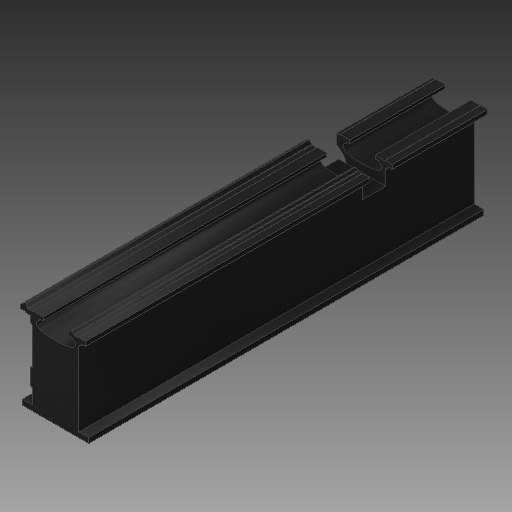
# Autodesk Inventor part: BED
Saved by Autodesk Inventor 2018 (Build 220112000, 112)
## iProperties
Created: 2017-02-14
Part Number: BED
Material: Iron, Cast
Document SubType Name: Modeling
Designer: M228540
Density: 7.15 g/cm^3
Appearance: Black Cast
Author: M228540
Autodesk Inventor part; units mm, degrees
ref_plane "YZ Plane" through (0, 0, 0) normal (1, 0, 0) x (0, 1, 0)
ref_plane "XZ Plane" through (0, 0, 0) normal (0, 1, 0) x (-1, 0, 0)
ref_plane "XY Plane" through (0, 0, 0) normal (0, 0, 1) x (1, 0, 0)
sketch "Sketch1" plane through (0, 0, 0) normal (0, 0, 1) x (1, 0, 0)
  line L0 (11.5989, 4.8072) -> (2.0726, 10.3072)
  line L1 (11.5989, 4.8072) -> (22.5989, 4.8072) construction
  line L2 (2.0726, 10.3072) -> (-7.9274, 10.3072)
  line L3 (-7.9274, 10.3072) -> (-7.9274, 22.0072)
  line L4 (-7.9274, 22.0072) -> (0.1717, 31.6594)
  line L5 (0.1717, 31.6594) -> (3.9717, 31.6594)
  line L6 (3.9717, 31.6594) -> (11.7854, 25.103)
  line L7 (11.7854, 25.103) -> (11.7854, 21.903)
  line L8 (11.7854, 21.903) -> (27.8854, 21.903)
  line L9 (27.8854, 21.903) -> (27.8854, 23.903)
  line L10 (27.8854, 23.903) -> (53.0854, 23.903)
  line L11 (53.0854, 23.903) -> (53.0854, 8.203)
  line L12 (53.0854, 8.203) -> (38.3854, 8.203)
  line L13 (38.3854, 8.203) -> (38.3854, 0.203) construction
  line L14 (38.3854, 0.203) -> (33.7666, 0.203) construction
  line L15 (38.3854, 8.203) -> (33.7666, 0.203)
  line L16 (38.3854, 8.203) -> (62.019, 8.203) construction
  line L17 (33.7666, 0.203) -> (33.7666, -3.797) construction
  arc A0 (33.7666, 0.203) -> (29.7666, -3.797) centre (33.7666, -3.797) ccw
  line L18 (29.7666, -3.797) -> (29.7666, -65.797)
  line L19 (29.7666, -65.797) -> (29.7666, -269.797)
  line L20 (-7.9274, 10.3072) -> (84.2692, 10.3072) construction
  line L21 (-100.122, 11.3032) -> (-98.5294, 23.903)
  line L22 (-98.5294, 23.903) -> (-134.7294, 23.903)
  line L23 (-98.5294, 23.903) -> (-62.3294, 23.903) construction
  line L24 (-134.7294, 23.903) -> (-134.7294, 21.903)
  line L25 (-134.7294, 21.903) -> (-153.7294, 21.903)
  line L26 (-153.7294, 21.903) -> (-153.7294, 23.903)
  line L27 (-153.7294, 23.903) -> (-162.2142, 34.0148)
  line L28 (-162.2142, 34.0148) -> (-166.8142, 34.0148)
  line L29 (-166.8142, 34.0148) -> (-179.0709, 23.7302)
  line L30 (-179.0709, 23.7302) -> (-179.0709, 9.7302)
  line L31 (-179.0709, 9.7302) -> (-165.0709, 9.7302)
  line L32 (-165.0709, 9.7302) -> (-165.0709, 6.7302) construction
  line L33 (-165.0709, 6.7302) -> (-163.3389, 6.7302) construction
  line L34 (-165.0709, 9.7302) -> (-163.3389, 6.7302)
  line L35 (-165.0709, 9.7302) -> (-161.6857, 9.7302) construction
  line L36 (-163.3389, 6.7302) -> (-145.9389, 6.7302)
  line L37 (-145.9389, 6.7302) -> (-145.9389, -15.7698)
  line L38 (-145.9389, -15.7698) -> (-145.9389, -22.7698) construction
  arc A1 (-138.9389, -22.7698) -> (-145.9389, -15.7698) centre (-145.9389, -22.7698) ccw
  line L39 (-138.9389, -22.7698) -> (-138.9389, -157.2698)
  line L40 (-138.9389, -22.7698) -> (-4.4389, -22.7698) construction
  line L41 (-138.9389, -157.2698) -> (-145.9389, -157.2698)
  line L42 (-145.9389, -157.2698) -> (-145.9389, -212.7698)
  line L43 (-145.9389, -212.7698) -> (-138.9389, -212.7698)
  line L44 (-138.9389, -212.7698) -> (-138.9389, -269.797)
  line L45 (-138.9389, -22.7698) -> (-145.9389, -22.7698) construction
  line L46 (29.7666, -3.797) -> (33.7666, -3.797) construction
  line L47 (-138.9389, -269.797) -> (-173.9389, -269.797)
  line L48 (-138.9389, -269.797) -> (-103.9389, -269.797) construction
  line L49 (-173.9389, -269.797) -> (-173.9389, -287.797)
  line L50 (29.7666, -269.797) -> (64.7666, -269.797)
  line L51 (29.7666, -269.797) -> (64.7666, -269.797) construction
  line L52 (64.7666, -269.797) -> (64.7666, -287.797)
  line L53 (64.7666, -287.797) -> (-173.9389, -287.797)
  line L54 (-100.122, 11.3032) -> (-110.722, 11.3032)
  line L55 (-100.122, 11.3032) -> (-89.522, 11.3032) construction
  line L56 (-110.722, 11.3032) -> (-114.722, 4.375)
  line L57 (-114.722, 4.375) -> (-119.5625, 1.8016) construction
  line L58 (-119.5625, 1.8016) -> (-124.3659, -3.6968) construction
  line L59 (-124.3659, -3.6968) -> (-125.2502, -13.8603) construction
  line L60 (-125.2502, -13.8603) -> (-112.722, -24.0101) construction
  line L61 (-112.722, -24.0101) -> (-52.4666, -30.3406) construction
  line L62 (-52.4666, -30.3406) -> (0.1681, -22.7698) construction
  line L63 (0.1681, -22.7698) -> (13.3927, -16.0523) construction
  line L64 (13.3927, -16.0523) -> (19.8318, -4.9385) construction
  line L65 (19.8318, -4.9385) -> (14.7145, 3.0084) construction
  line L66 (14.7145, 3.0084) -> (11.5989, 4.8072) construction
  spline S0 degree 4 poles (-114.722, 4.375) (-119.5625, 1.8016) (-124.3659, -3.6968) (-125.2502, -13.8603) (-112.722, -24.0101) (-52.4666, -30.3406) (0.1681, -22.7698) (13.3927, -16.0523) (19.8318, -4.9385) (14.7145, 3.0084) (11.5989, 4.8072) knots 0 0 0 0 0 1 2 3 4 5 6 7 7 7 7 7
  point P0 (0, 0)
  dimension "d0" = 11
  dimension "d1" = 150
  dimension "d2" = 10
  dimension "d3" = 11.7
  dimension "d4" = 12.6
  dimension "d5" = 140
  dimension "d6" = 3.8
  dimension "d7" = 10.2
  dimension "d8" = 140
  dimension "d9" = 3.2
  dimension "d10" = 16.1
  dimension "d11" = 2
  dimension "d12" = 25.2
  dimension "d13" = 15.7
  dimension "d14" = 14.7
  dimension "d15" = 8
  dimension "d16" = 120
  dimension "d17" = 4
  dimension "d18" = 62
  dimension "d19" = 204
  dimension "d22" = 92.2
  dimension "d24" = 12.7
  dimension "d25" = 36.2
  dimension "d26" = 180
  dimension "d27" = 2
  dimension "d28" = 19
  dimension "d29" = 2
  dimension "d30" = 13.2
  dimension "d31" = 140
  dimension "d32" = 4.6
  dimension "d33" = 16
  dimension "d34" = 140
  dimension "d35" = 14
  dimension "d36" = 14
  dimension "d37" = 90
  dimension "d38" = 3
  dimension "d39" = 60
  dimension "d40" = 17.4
  dimension "d41" = 22.5
  dimension "d43" = 134.5
  dimension "d44" = 90
  dimension "d46" = 55.5
  dimension "d47" = 90
  dimension "d50" = 90
  dimension "d51" = 35
  dimension "d52" = 180
  dimension "d53" = 18
  dimension "d54" = 90
  dimension "d55" = 35
  dimension "d57" = 18
  dimension "d59" = 180
  dimension "d60" = 8
  dimension "d61" = 120
  dimension "d62" = 62
  dimension "d98" = 7
  dimension "d103" = 7
  constraints: 114 end point, 22 perpendicular, 19 horizontal, 6 equal length, 5 vertical, 4 point on circle, 4 point on line, 2 centre point, 2 coincident, 2 parallel, 1 collinear, 3 other
  measures "d0" distance of L0.start L0.end
  measures "d1" angle of L1 L0
  measures "d2" distance of L0.end L2.end
  measures "d3" distance of L2.end L3.end
  measures "d4" distance of L3.end L4.end
  measures "d5" angle of L3 L4
  measures "d6" distance of L4.end L5.end
  measures "d7" distance of L5.end L6.end
  measures "d8" angle of L5 L6
  measures "d9" distance of L6.end L7.end
  measures "d10" distance of L7.end L8.end
  measures "d11" distance of L8.end L9.end
  measures "d12" distance of L9.end L10.end
  measures "d13" distance of L10.end L11.end
  measures "d14" distance of L11.end L12.end
  measures "d15" distance of L12.end L13.end
  measures "d16" angle of L15 L16
  measures "d17" distance of L14.end L17.end
  measures "d18" distance of L18.start L18.end
  measures "d19" distance of L18.end L19.end
  measures "d22" distance of L2.end L21.start
  measures "d24" distance of L21.start L21.end
  measures "d25" distance of L21.end L22.end
  measures "d26" angle of L22 L23
  measures "d27" distance of L22.end L24.end
  measures "d28" distance of L24.end L25.end
  measures "d29" distance of L25.end L26.end
  measures "d30" distance of L26.end L27.end
  measures "d31" angle of L27 L26
  measures "d32" distance of L27.end L28.end
  measures "d33" distance of L28.end L29.end
  measures "d34" angle of L29 L28
  measures "d35" distance of L29.end L30.end
  measures "d36" distance of L30.end L31.end
  measures "d37" angle of L31 L30
  measures "d38" distance of L31.end L32.end
  measures "d39" angle of L34 L35
  measures "d40" distance of L33.end L36.end
  measures "d41" distance of L36.end L37.end
  measures "d43" distance of L39.start L39.end
  measures "d44" angle of L39 L40
  measures "d46" distance of L41.end L42.end
  measures "d47" angle of L42 L41
  measures "d50" angle of L43 L44
  measures "d51" distance of L44.end L47.end
  measures "d52" angle of L47 L48
  measures "d53" distance of L47.end L49.end
  measures "d54" angle of L49 L47
  measures "d55" distance of L19.end L50.end
  measures "d57" distance of L50.end L52.end
  measures "d59" angle of L54 L55
  measures "d60" distance of L54.end L56.end
  measures "d61" angle of L56 L54
  measures "d62" distance from line of L5 L61.end
  measures "d98" radius of A1
  measures "d103" distance of L39.end L41.end
extrude "Extrusion1" add sketch "Sketch1" against normal blind 1420
chamfer "Chamfer1" distance 4 angle 45 2 edges at (-138.9389, -157.2698, -710) (-138.9389, -212.7698, -710)
ref_plane "Work Plane3" through (-62.9928, 23.7302, -1420) normal (-1, 0, 0) x (0, 0, 1)
sketch "Sketch2" plane through (-62.9928, 23.7302, -1420) normal (-1, 0, 0) x (0, 0, 1)
  line L0 (1420, 7.9292) -> (0, 7.9292) projected
  line L1 (400, 7.9292) -> (400, -79.7708)
  line L2 (400, -79.7708) -> (318, -79.7708)
  line L3 (318, -79.7708) -> (318, 139.9542)
  line L4 (1420, -27.5272) -> (0, -27.5272) projected
  line L5 (318, 139.9542) -> (400, 139.9542)
  line L6 (400, 139.9542) -> (400, 7.9292)
  line L7 (1420, -27.5272) -> (1420, -293.5272) projected
  point P0 (1420, -23.7302)
  dimension "d68" = 1020
  dimension "d69" = 82
  dimension "d70" = 87.7
  constraints: 10 end point, 4 perpendicular, 2 point on line, 1 vertical
  measures "d68" distance between parallel lines of L7 L1
  measures "d69" distance of L1.end L2.end
  measures "d70" distance between parallel lines of L2 L0
extrude "Extrusion2" cut sketch "Sketch2" along normal through all both and the other way through all
sketch "Sketch3" plane through (0, 0, -1420) normal (0, 0, -1) x (-1, 0, 0)
  line L0 (-11.7854, 21.903) -> (13.84, 21.903)
  line L1 (13.84, 21.903) -> (13.84, 35.1766)
  line L2 (13.84, 35.1766) -> (-11.7854, 35.1766)
  line L3 (-11.7854, 25.103) -> (-11.7854, 21.903) projected
  line L4 (-11.7854, 35.1766) -> (-11.7854, 21.903)
  point P0 (0, 0)
  constraints: 8 end point, 2 perpendicular, 1 collinear, 1 horizontal
extrude "Extrusion3" cut sketch "Sketch3" against normal up to surface (318 mm away)
sketch "Sketch4" plane through (0, 0, -1420) normal (0, 0, -1) x (-1, 0, 0)
  line L0 (163.3389, 6.7302) -> (145.9389, 6.7302) projected
  line L1 (145.9389, 6.7302) -> (145.9389, 38.3336)
  line L2 (145.9389, 38.3336) -> (189.5929, 38.3336)
  line L3 (189.5929, 38.3336) -> (189.5929, 6.7302)
  line L4 (189.5929, 6.7302) -> (145.9389, 6.7302)
  point P0 (0, 0)
  constraints: 8 end point, 2 perpendicular, 1 collinear, 1 vertical
extrude "Extrusion4" cut sketch "Sketch4" against normal up to surface (318 mm away)
sketch "Sketch5" plane through (0, 0, -1420) normal (0, 0, -1) x (-1, 0, 0)
  arc A0 (145.9389, -15.7698) -> (138.9389, -22.7698) centre (145.9389, -22.7698) ccw projected
  line L0 (142.5187, -16.6623) -> (135.4261, -21.5718) construction
  line L1 (135.4261, -21.5718) -> (129.175, -25.2698) construction
  line L2 (129.175, -25.2698) -> (115.3794, -37.954) construction
  line L3 (115.3794, -37.954) -> (107.9389, -59.7698) construction
  line L4 (107.9389, -59.7698) -> (111.1778, -81.5318) construction
  line L5 (111.1778, -81.5318) -> (116.1934, -117.4769) construction
  line L6 (116.1934, -117.4769) -> (138.9389, -184.797) construction
  spline S0 degree 4 poles (142.5187, -16.6623) (135.4261, -21.5718) (129.175, -25.2698) (115.3794, -37.954) (107.9389, -59.7698) (111.1778, -81.5318) (116.1934, -117.4769) (138.9389, -184.797) knots 1 1 1 1 1 2 3 4 5 5 5 5 5
  line L7 (173.9389, -269.797) -> (138.9389, -269.797) projected
  line L8 (138.9389, -153.2698) -> (138.9389, -22.7698) projected
  line L9 (138.9389, -269.797) -> (138.9389, -216.7698) projected
  line L10 (138.9389, -184.797) -> (138.9389, -216.7698)
  line L11 (138.9389, -216.7698) -> (164.8959, -216.7698)
  line L12 (164.8959, -216.7698) -> (151.2972, -16.0675)
  line L13 (151.2972, -16.0675) -> (142.5187, -16.6623)
  point P0 (0, 0)
  point P1 (141.8818, -156.5627)
  point P2 (141.8818, -211.9923)
  dimension "d77" = 85
  dimension "d78" = 31
  dimension "d79" = 44
  constraints: 8 end point, 2 perpendicular, 1 point on circle, 1 vertical, 5 other
  measures "d77" distance from line of L7 L6.end
  measures "d79" vertical distance of A0.start L3.end
extrude "Extrusion5" cut sketch "Sketch5" against normal up to surface (318 mm away) contours L13 L12 L11 L10 S0
sketch "Sketch6" plane through (0, 0, -1420) normal (0, 0, -1) x (-1, 0, 0)
  line L0 (145.9389, 21.903) -> (134.7294, 21.903) projected
  line L1 (134.7294, 21.903) -> (134.7294, 23.903) projected
  line L2 (134.7294, 23.903) -> (98.5294, 23.903) projected
  line L3 (98.5294, 23.903) -> (100.122, 11.3032) projected
  line L4 (100.122, 11.3032) -> (110.722, 11.3032) projected
  line L5 (110.722, 11.3032) -> (114.722, 4.375) projected
  spline S0 degree 4 poles (114.722, 4.375) (119.5625, 1.8016) (124.3659, -3.6968) (125.2502, -13.8603) (112.722, -24.0101) (52.4666, -30.3406) (-0.1681, -22.7698) (-13.3927, -16.0523) (-19.8318, -4.9385) (-14.7145, 3.0084) (-11.5989, 4.8072) knots 0 0 0 0 0 0.142857 0.285714 0.428571 0.571429 0.714286 0.857143 1 1 1 1 1 projected
  line L6 (145.9389, -15.7698) -> (145.9389, 21.903) projected
  line L7 (-11.5989, 4.8072) -> (-2.0726, 10.3072) projected
  line L8 (-2.0726, 10.3072) -> (7.9274, 10.3072) projected
  line L9 (7.9274, 10.3072) -> (7.9274, 21.903) projected
  line L10 (7.9274, 21.903) -> (-27.8854, 21.903) projected
  line L11 (-27.8854, 23.903) -> (-53.0854, 23.903) projected
  line L12 (-27.8854, 21.903) -> (-27.8854, 23.903) projected
  line L13 (-53.0854, 23.903) -> (-53.0854, 8.203) projected
  line L14 (-53.0854, 8.203) -> (-38.3854, 8.203) projected
  line L15 (-38.3854, 8.203) -> (-33.7666, 0.203) projected
  arc A0 (-29.7666, -3.797) -> (-33.7666, 0.203) centre (-33.7666, -3.797) ccw projected
  line L16 (-33.7666, 0.203) -> (-15.75, 0.203)
  line L17 (120.3191, 0.203) -> (145.9389, 0.203)
  point P0 (0, 0)
  constraints: 4 end point, 2 perpendicular, 2 tangent, 1 point on line, 3 other
extrude "Extrusion6" add sketch "Sketch6" along normal blind 26
sketch "Sketch8" plane through (-145.9389, -15.7698, 0) normal (-1, 0, 0) x (0, 0, 1)
  circle A0 centre (-32.5, 9.5) radius 4
  circle A1 centre (-18.5, 9.5) radius 4
  line L0 (0, 0) -> (0, 22.5) projected
  line L1 (0, 22.5) -> (-1020, 22.5) projected
  point P0 (0, 15.7698)
  dimension "d84" = 8
  dimension "d85" = 8
  dimension "d86" = 18.5
  dimension "d87" = 14
  dimension "d88" = 13
  constraints: 2 centre point, 1 horizontal alignment
  measures "d84" diameter of A1
  measures "d85" diameter of A0
  measures "d86" distance from line of L0 A1.centre
  measures "d87" distance of A1.centre A0.centre
  measures "d88" distance from line of L1 A1.centre
extrude "Extrusion7" cut sketch "Sketch8" against normal blind 10
sketch "Sketch9" plane through (-145.9389, -212.7698, 0) normal (-1, 0, 0) x (0, 0, 1)
  circle A0 centre (-36.5, 34.5) radius 4
  circle A1 centre (-22.5, 34.5) radius 4
  circle A2 centre (-18.5, 206.5) radius 4 projected
  line L0 (0, 0) -> (0, 55.5) projected
  point P0 (0, 212.7698)
  dimension "d91" = 8
  dimension "d92" = 8
  dimension "d93" = 172
  dimension "d94" = 22.5
  dimension "d95" = 14
  constraints: 2 centre point, 1 horizontal alignment
  measures "d91" diameter of A0
  measures "d92" diameter of A1
  measures "d93" vertical distance of A1.centre A2.centre
  measures "d94" distance from line of A1.centre L0
  measures "d95" distance of A1.centre A0.centre
extrude "Extrusion8" cut sketch "Sketch9" against normal blind 20 contours A0 | A1
ref_plane "Work Plane4" through (-110.9735, -56.0406, -1242) normal (0, 0, -1) x (-1, 0, 0)
ref_plane "Work Plane5" through (-110.9735, -56.0406, -1292) normal (0, 0, -1) x (-1, 0, 0)
sketch "Sketch10" plane through (-110.9735, -56.0406, -1102) normal (0, 0, -1) x (-1, 0, 0)
  line L0 (27.9654, -128.7564) -> (34.9654, -128.7564)
  line L1 (34.9654, -101.2292) -> (34.9654, -156.7292) projected
  line L2 (34.9654, -128.7564) -> (34.9654, -156.7292)
  line L3 (34.9654, -156.7292) -> (27.9654, -160.7292)
  line L4 (27.9654, -160.7292) -> (27.9654, -128.7564)
  line L5 (27.9654, -160.7292) -> (27.9654, -128.7564) projected
  point P0 (-110.9735, 56.0406)
  constraints: 8 end point, 2 collinear, 1 horizontal, 1 point on line
extrude "Extrusion9" add sketch "Sketch10" along normal up to surface (50 mm away) from surface at 140
sketch "Sketch11" plane through (-138.9389, -153.2698, 0) normal (-1, 0, 0) x (0, 0, 1)
  line L0 (0, 130.5) -> (0, 137.5) projected
  line L1 (0, 0) -> (-1102, 0) projected
  line L2 (0, 130.5) -> (-40, 130.5)
  line L3 (-40, 130.5) -> (-40, 0)
  line L4 (-40, 0) -> (0, 0)
  line L5 (0, 0) -> (0, 130.5)
  line L6 (0, 0) -> (0, 130.5) projected
  point P0 (0, 153.2698)
  dimension "d104" = 40
  constraints: 8 end point, 2 parallel, 1 horizontal, 1 perpendicular, 1 point on line
  measures "d104" distance between parallel lines of L6 L3
extrude "Extrusion10" cut sketch "Sketch11" against normal blind 2
sketch "Sketch12" plane through (-145.9389, -212.7698, -1292) normal (-1, 0, 0) x (0, 0, 1)
  circle A0 centre (23, 12.6728) radius 4 projected
  circle A1 centre (40, 214.6728) radius 4 projected
  circle A2 centre (100, 214.6728) radius 4 projected
  circle A3 centre (160, 214.6728) radius 4 projected
  circle A4 centre (213, 14.6728) radius 4 projected
  circle A5 centre (253, 34.6728) radius 4 projected
  point P0 (1292, 212.7698)
extrude "Extrusion11" cut sketch "Sketch12" against normal blind 20
body "Solid1"
